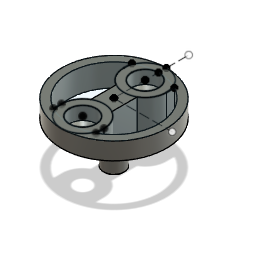
MagnetHolder (Autodesk Fusion 360 design; units mm, degrees)
Autodesk Fusion 360 part; units mm, degrees
note: some values were not read from the file. Chosen so that the rebuilt part matches the saved one: where a step ends; which pieces of a blend or face edit are solid.
sketch "Skizze1" plane through (0, 0, 0) normal (0, 1, 0) x (1, 0, 0)
  circle A0 centre (0, 0) radius 4
  circle A1 centre (0, 0) radius 1.1
  dimension "d1" = 8
  dimension "d2" = 2.2
  constraint coincident A0.centre A1.centre
  constraint concentric A0 A1
  measures "d1" diameter of A0
  measures "d2" diameter of A1
extrude "Extrusion1" add sketch "Skizze1" along normal blind 6.68 contours A0 picked at (3.018441, -0.198723) makes body 1
sketch "Skizze2" plane through (0, 0, 0) normal (1, 0, 0) x (0, 0, -1)
  line L0 (-1.1, 6.68) -> (1.1, 6.68)
  line L1 (4, 6.68) -> (-4, 6.68)
  line L2 (-4, 6.68) -> (-20, 17.883321) construction
  line L3 (0, 0) -> (0, 54.133053) construction
  line L4 (-20, 17.883321) -> (-20, 22.8133)
  line L5 (-20, 22.8133) -> (-17, 22.8133)
  line L6 (-17, 22.8133) -> (-17, 17.8133)
  line L7 (-17, 17.8133) -> (-1.1, 6.68)
  line L8 (4, 6.68) -> (-4, 6.68)
  line L9 (4, 0) -> (-4, 0)
  line L10 (-4, 6.68) -> (-4, 0) construction
  line L11 (-4, 5.048278) -> (-20, 16.251599)
  line L12 (-20, 16.251599) -> (-20, 17.883321)
  line L13 (-4, 5.048278) -> (-4, 6.68)
  line L14 (-1.1, 6.68) -> (-4, 6.68)
  dimension "d8" = 55
  dimension "d9" = 20
  dimension "d10" = 3
  dimension "d11" = 3
  dimension "d12" = 5
  constraint coincident L1.end L2.start
  constraint coincident L3.start origin
  constraint perpendicular L0 L3
  constraint vertical L4
  constraint perpendicular L4 L5
  constraint perpendicular L5 L6
  constraint coincident L0.start L7.end
  constraint parallel L2 L7
  constraint coincident L9.end L10.end
  constraint parallel L2 L11
  constraint vertical L12
  measures "d8" angle of L2 L3
  measures "d10" distance of L4 L6
  measures "d11" distance of L7 L11
  measures "d12" distance of L5.end L6.end
revolve "Drehen1" add sketch "Skizze2" angle 360 about axis through (0, 0, 0) along (0, 1, 0) contours L1 L4 L5 L6 L7 L8 L11 L12 L13 L14 picked at (-13.666667, 13.581633) bodies 1
sketch "Skizze3" plane through (0, 22.8133, 0) normal (0, 1, 0) x (-1, 0, 0)
  circle A0 centre (0, 0) radius 20
  circle A1 centre (0, 0) radius 17
  line L0 (0, 0) -> (0, -28.536581) construction
  circle A2 centre (0, -11.9) radius 5.1
  circle A3 centre (0, -11.9) radius 8.1
  line L1 (0, 0) -> (-22.216074, 0) construction
  line L2 (8.1, -11.9) -> (8.1, -14.946237)
  line L3 (-8.1, -11.9) -> (-8.1, -14.946237)
  circle A4 centre (0, 11.9) radius 8.1
  circle A5 centre (0, 11.9) radius 5.1
  line L4 (-8.1, 11.9) -> (-8.1, 14.946237)
  line L5 (8.1, 11.9) -> (8.1, 14.946237)
  point P0 (0, -17)
  point P1 (0, -20)
  dimension "d15" = 10.2
  constraint coincident A0.centre A1.centre
  constraint vertical L0
  constraint coincident A1 P0
  constraint coincident L0 P0
  constraint coincident L0 A2.centre
  constraint coincident P0 A2
  constraint concentric A2 A3
  constraint coincident L0 P1
  constraint coincident A0 P1
  constraint coincident A3 P1
  constraint perpendicular L0 L1
  constraint coincident A3 L2.start
  constraint vertical L2
  constraint coincident A3 L3.start
  constraint vertical L3
  constraint tangent A3 L3
  constraint tangent A3 L2
  constraint symmetric A2 L1 A5
  constraint symmetric A3 L1 A4
  constraint symmetric L1 L2.start L5.start
  constraint symmetric L1 L3.start L4.start
  measures "d15" diameter of A2
extrude "Extrusion2" add sketch "Skizze3" along normal up to near side of body 1 contours A5 | A1 A4 | A1 A4 L5 | A1 A4 L4 | A2 | A1 A3 | A1 A3 L3 | A1 A3 L2 picked at (0.969475, 12.535052) picked at (-5.995386, 15.03885) picked at (7.956923, 14.085703) picked at (-7.956923, 14.085703) picked at (-0.460937, -13.690423) picked at (-5.995386, -15.03885) picked at (-7.956923, -14.085703) picked at (7.956923, -14.085703) bodies 1
extrude "Extrusion3" cut sketch "Skizze3" along normal up to surface contours A5 | A2 picked at (0.969475, 12.535052) picked at (-0.460937, -13.690423) end surface at (-14.241307, 13.761972, 8.222222) on bodies 1 bodies 1
ref_plane "Arbeitsebene1" through (0, 17.8133, 11.9) normal (0, 1, 0) x (-1, 0, 0)
sketch "Skizze4" plane through (0, 17.8133, 12) normal (0, 1, 0) x (1, 0, 0)
  circle A0 centre (0, 0.1) radius 5.1
  circle A1 centre (0, 0.1) radius 3.1
  dimension "d21" = -2
extrude "Extrusion4" add sketch "Skizze4" against normal blind 3 contours A0 picked at (4.402804, -0.307382) bodies 1
ref_plane "Arbeitsebene2" through (0, 16.3133, 11.9) normal (0, 0, 1) x (0, -1, 0)
sketch "Skizze5" plane through (0, 16.383321, 11.9) normal (0, 0, 1) x (1, 0, 0)
  line L0 (3.1, -1.570021) -> (-3.1, -1.570021)
  line L1 (-3.1, 1.429979) -> (3.1, 1.429979)
  line L2 (-3.1, 1.429979) -> (3.1, 1.429979)
  line L3 (-5.1, 1.429979) -> (5.1, 1.429979)
  line L4 (3.1, -1.570021) -> (3.1, 1.429979) construction
  line L5 (3.1, 1.429979) -> (5.1, 1.429979)
  line L6 (5.1, 1.429979) -> (3.1, 0.029564)
  line L7 (3.1, 0.029564) -> (3.1, 1.429979)
  dimension "d25" = 35
  constraint perpendicular L3 L7
  measures "d25" angle of L5 L6
revolve "Drehen2" cut sketch "Skizze5" angle 360 about axis through (0, 19.3133, 11.9) along (0, -1, 0) contours L3 L5 L6 L7 picked at (3.766667, 0.963174) bodies 1
sketch "Skizze6" plane through (0, 0, 0) normal (1, 0, 0) x (0, 0, -1)
  spline S0 degree 3 poles (-9.714286, 9.7759) (-9.28231, 9.441124) (-8.843075, 9.076326) (-8.067061, 8.377565) (-7.730039, 8.043745) (-7.278279, 7.566701) (-7.10138, 7.366776) (-6.861836, 7.086073) (-6.8, 7.008859) (-6.8, 7.008859) (-6.861836, 7.086073) (-7.10138, 7.366776) (-7.278279, 7.566701) (-7.730039, 8.043745) (-8.067061, 8.377565) (-8.843075, 9.076326) (-9.28231, 9.441124) (-10.432862, 10.332788) (-11.284279, 10.924737) (-13.009067, 12.015854) (-13.881113, 12.517096) (-14.962753, 13.108174) (-15.309007, 13.292239) (-15.922205, 13.611548) (-16.188744, 13.74692) (-16.576072, 13.941714) (-16.737299, 14.021627) (-16.949361, 14.126245) (-17, 14.150976) (-17, 14.150976) (-16.949361, 14.126245) (-16.737299, 14.021627) (-16.576072, 13.941714) (-16.188744, 13.74692) (-15.922205, 13.611548) (-15.309007, 13.292239) (-14.962753, 13.108174) (-13.881113, 12.517096) (-13.009067, 12.015854) (-11.284279, 10.924737) (-10.432862, 10.332788) (-9.714286, 9.7759) knots 0 0 0 0 0.17509934 0.17509934 0.35019868 0.35019868 0.48325281 0.48325281 0.61630694 0.61630694 0.74936107 0.74936107 0.8824152 0.8824152 1.05751454 1.05751454 1.23261388 1.23261388 1.5238853 1.5238853 1.81515672 1.81515672 1.94679969 1.94679969 2.07844266 2.07844266 2.19887566 2.19887566 2.31930865 2.31930865 2.43974165 2.43974165 2.56017465 2.56017465 2.69181762 2.69181762 2.82346058 2.82346058 3.114732 3.114732 3.40600342 3.40600342 3.40600342 3.40600342
  line L0 (-6.8, 14.8133) -> (-17, 14.8133)
  spline S1 degree 3 poles (-9.714286, 9.7759) (-9.28231, 9.441124) (-8.843075, 9.076326) (-8.067061, 8.377565) (-7.730039, 8.043745) (-7.278279, 7.566701) (-7.10138, 7.366776) (-6.861836, 7.086073) (-6.8, 7.008859) (-6.8, 7.008859) (-6.861836, 7.086073) (-7.10138, 7.366776) (-7.278279, 7.566701) (-7.730039, 8.043745) (-8.067061, 8.377565) (-8.843075, 9.076326) (-9.28231, 9.441124) (-10.432862, 10.332788) (-11.284279, 10.924737) (-13.009067, 12.015854) (-13.881113, 12.517096) (-14.962753, 13.108174) (-15.309007, 13.292239) (-15.922205, 13.611548) (-16.188744, 13.74692) (-16.576072, 13.941714) (-16.737299, 14.021627) (-16.949361, 14.126245) (-17, 14.150976) (-17, 14.150976) (-16.949361, 14.126245) (-16.737299, 14.021627) (-16.576072, 13.941714) (-16.188744, 13.74692) (-15.922205, 13.611548) (-15.309007, 13.292239) (-14.962753, 13.108174) (-13.881113, 12.517096) (-13.009067, 12.015854) (-11.284279, 10.924737) (-10.432862, 10.332788) (-9.714286, 9.7759) knots 0 0 0 0 0.17509934 0.17509934 0.35019868 0.35019868 0.48325281 0.48325281 0.61630694 0.61630694 0.74936107 0.74936107 0.8824152 0.8824152 1.05751454 1.05751454 1.23261388 1.23261388 1.5238853 1.5238853 1.81515672 1.81515672 1.94679969 1.94679969 2.07844266 2.07844266 2.19887566 2.19887566 2.31930865 2.31930865 2.43974165 2.43974165 2.56017465 2.56017465 2.69181762 2.69181762 2.82346058 2.82346058 3.114732 3.114732 3.40600342 3.40600342 3.40600342 3.40600342
  spline S2 degree 3 poles (9.714286, 9.7759) (9.28231, 9.441124) (8.843075, 9.076326) (8.067061, 8.377565) (7.730039, 8.043745) (7.278279, 7.566701) (7.10138, 7.366776) (6.861836, 7.086073) (6.8, 7.008859) (6.8, 7.008859) (6.861836, 7.086073) (7.10138, 7.366776) (7.278279, 7.566701) (7.730039, 8.043745) (8.067061, 8.377565) (8.843075, 9.076326) (9.28231, 9.441124) (10.432862, 10.332788) (11.284279, 10.924737) (13.009067, 12.015854) (13.881113, 12.517096) (14.962753, 13.108174) (15.309007, 13.292239) (15.922205, 13.611548) (16.188744, 13.74692) (16.576072, 13.941714) (16.737299, 14.021627) (16.949361, 14.126245) (17, 14.150976) (17, 14.150976) (16.949361, 14.126245) (16.737299, 14.021627) (16.576072, 13.941714) (16.188744, 13.74692) (15.922205, 13.611548) (15.309007, 13.292239) (14.962753, 13.108174) (13.881113, 12.517096) (13.009067, 12.015854) (11.284279, 10.924737) (10.432862, 10.332788) (9.714286, 9.7759) knots 0 0 0 0 0.17509934 0.17509934 0.35019868 0.35019868 0.48325281 0.48325281 0.61630694 0.61630694 0.74936107 0.74936107 0.8824152 0.8824152 1.05751454 1.05751454 1.23261388 1.23261388 1.5238853 1.5238853 1.81515672 1.81515672 1.94679969 1.94679969 2.07844266 2.07844266 2.19887566 2.19887566 2.31930865 2.31930865 2.43974165 2.43974165 2.56017465 2.56017465 2.69181762 2.69181762 2.82346058 2.82346058 3.114732 3.114732 3.40600342 3.40600342 3.40600342 3.40600342
  line L1 (-4, 5.048278) -> (4, 5.048278)
  line L2 (20, 16.251599) -> (-20, 16.251599)
  line L3 (-4, 5.048278) -> (-20, 16.251599) construction
  line L4 (-17, 14.8133) -> (-17, 14.150976)
  line L5 (-17, 14.150976) -> (-6.8, 7.008859)
  line L6 (-6.8, 14.8133) -> (-6.8, 7.008859)
  line L7 (-17, 14.8133) -> (-6.8, 14.8133)
  constraint coincident L0.end L4.start
  constraint perpendicular L0 L4
  constraint coincident L0.start L6.start
  constraint vertical L6
revolve "Drehen3" add sketch "Skizze6" angle 30 about axis through (0, 1.75, 0) along (0, 1, 0) second angle 30 contours S0 L0 S1 L4 L6 L7 | S0 S1 L5 picked at (-9.451624, 11.95454) picked at (-12.706252, 11.304895) bodies 1
extrude "Extrusion5" cut 1 faces at (0.861796, 14.8133, 11.85772) along direction (0, 1, 0) up to surface end surface at (7.111341, 14.056, -15.291679) on bodies 1 bodies 1
mirror "Spiegeln2" about plane through (0, 0, 0) normal (0, 0, 1) of "Extrusion4", "Drehen2", "Drehen3", "Extrusion5"
sketch "Skizze7" plane through (0, 22.8133, 0) normal (0, 1, 0) x (-1, 0, 0)
  circle A0 centre (0, 11.9) radius 5.1
  circle A1 centre (0, -11.9) radius 5.1
  circle A2 centre (0, 0) radius 20
  arc A3 (8.1, -14.946237) -> (8.1, 14.946237) centre (0, 0) ccw
  line L0 (8.1, -14.946237) -> (8.1, -11.9)
  arc A4 (8.1, -11.9) -> (-8.1, -11.9) centre (0, -11.9) ccw
  line L1 (-8.1, -11.9) -> (-8.1, -14.946237)
  arc A5 (-8.1, 14.946237) -> (-8.1, -14.946237) centre (0, 0) ccw
  line L2 (-8.1, 14.946237) -> (-8.1, 11.9)
  arc A6 (-8.1, 11.9) -> (8.1, 11.9) centre (0, 11.9) ccw
  line L3 (8.1, 11.9) -> (8.1, 14.946237)
  arc A7 (8.1, -11.9) -> (-8.1, -11.9) centre (0, -11.9) ccw
  line L4 (8.1, -11.9) -> (8.1, -14.946237)
  arc A8 (8.1, -14.946237) -> (8.1, 14.946237) centre (0, 0) ccw
  line L5 (-8.1, -11.9) -> (-8.1, -14.946237)
  arc A9 (-8.1, 14.946237) -> (-8.1, -14.946237) centre (0, 0) ccw
  line L6 (-8.1, 11.9) -> (-8.1, 14.946237)
  arc A10 (-8.1, 11.9) -> (8.1, 11.9) centre (0, 11.9) ccw
  line L7 (8.1, 11.9) -> (8.1, 14.946237)
  circle A11 centre (0, 0) radius 4
  line L8 (-4, -4.856563) -> (-4, 4.856563)
  line L9 (4, -4.856563) -> (4, 4.856563)
  circle A12 centre (0, 0) radius 1.1
  constraint vertical L8
  constraint vertical L9
  constraint tangent A11 L9
  constraint tangent A11 L8
extrude "Extrusion6" cut sketch "Skizze7" along normal up to surface contours A3 L0 A4 A6 L3 A7 L4 A8 A10 L7 L9 | A4 L1 A5 L2 A6 A7 L5 A9 L6 A10 L8 picked at (8.768712, 3.255359) picked at (-8.768712, -3.255359) end surface at (7.062401, 13.980792, 15.195984) on bodies 1 bodies 1
extrude "Extrusion7" add sketch "Skizze7" along normal up to surface contours A4 A7 A11 L9 | A6 A10 A11 L9 | A4 A7 A11 | A4 A6 A7 A10 A11 | A6 A10 A11 | A4 A7 A11 L8 | A6 A10 A11 L8 picked at (3.346894, -3.972334) picked at (3.346894, 3.972334) picked at (0, -3.871528) picked at (0.027401, -2.903836) picked at (0, 3.871528) picked at (-3.346894, -3.972334) picked at (-3.346894, 3.972334) end surface at (-2.263044, 8.625012, -3.148919) on bodies 1 bodies 1
chamfer "Fase1" distance 0.5 angle 45 2 edges at (-3.729309, 0, 1.446462) (-1.02556, 0, -0.397777) on bodies 1
sketch "Skizze8" plane through (-4, 0, 0) normal (-1, 0, 0) x (0, 0, 1)
  line L0 (-4.856563, 22.8133) -> (-4.856563, 6.652984)
  spline S0 degree 2 poles (0, 5.048278) (-1.887555, 5.048278) (-4.856563, 6.652984) knots 2.26925326 2.26925326 2.26925326 3.27118797 3.27118797 3.27118797 weights 1 1.32321959 1.36101936
  spline S1 degree 2 poles (4.856563, 6.652984) (1.887555, 5.048278) (0, 5.048278) knots 1.26731855 1.26731855 1.26731855 2.26925326 2.26925326 2.26925326 weights 1.36101936 1.32321959 1
  line L1 (4.856563, 6.652984) -> (4.856563, 22.8133)
  line L2 (4.856563, 22.8133) -> (-4.856563, 22.8133)
copy_body "Körper->Berechn1" bodies 1 removing the originals makes body 2 in component "MagnetHolder"
component "MagnetHolder" placed x (1, 0, 0) y (0, 1, 0) z (0, 0, 1) at (0, 0, 0)
equation "d2 = 2 mm + shaft_clearance"
equation "shaft_clearance = 0.2 mm"
equation "clearance = 0.32 mm"
equation "d5 = 7 mm - clearance"
equation "shaft_length = 7 mm"
equation "magnet_clearance = 0.2 mm"
equation "d15 = 10 mm + magnet_clearance"
